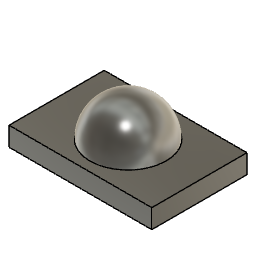
3D_manufacturing_parallel_25_min (Autodesk Fusion 360 design; units mm, degrees)
Autodesk Fusion 360 part; units mm, degrees
sketch "Sketch1" plane through (0, 0, 0) normal (0, 0, 1) x (1, 0, 0)
  line L0 (-75, 50) -> (75, 50)
  line L1 (75, 50) -> (75, -50)
  line L2 (75, -50) -> (-75, -50)
  line L3 (-75, -50) -> (-75, 50)
  line L4 (-75, 50) -> (75, -50) construction
  line L5 (75, 50) -> (-75, -50) construction
  dimension "d1" = 150
  dimension "d2" = 100
  constraint horizontal L0
  constraint perpendicular L0 L1
  constraint parallel L0 L2
  constraint parallel L1 L3
  constraint coincident L4 origin
  constraint coincident L5 origin
  measures "d1" distance of L0.start L0.end
  measures "d2" distance of L0.start L2.end
extrude "Extrude1" add sketch "Sketch1" along normal blind 20
sketch "Sketch2" plane through (0, 0, 20) normal (0, 0, 1) x (-1, 0, 0)
  line L0 (75, 50) -> (-75, 50)
  line L1 (-75, 50) -> (-75, -50)
  line L2 (-75, -50) -> (75, -50)
  line L3 (75, -50) -> (75, 50)
  circle A0 centre (0, 0) radius 40
  dimension "d5" = 80
  constraint coincident A0.centre origin
  measures "d5" diameter of A0
extrude "Extrude2" add sketch "Sketch2" along normal blind 40 contours A0
fillet "Fillet1" radius 40 1 edges at (37.2931, 14.4646, 60)
